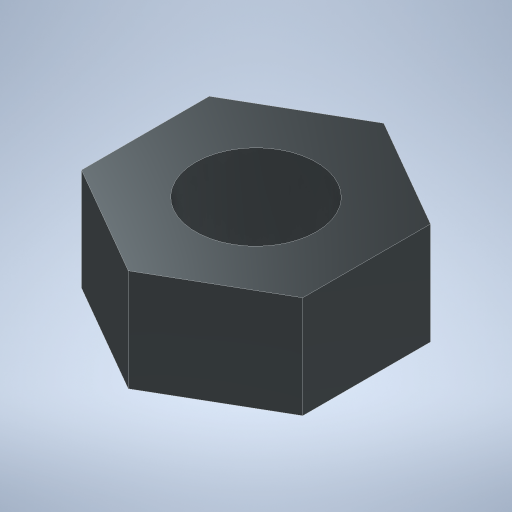
# Autodesk Inventor part: Threaded Rod nut
Saved by Autodesk Inventor 2024 (Build 280153000, 153)
## iProperties
Created: 2023-06-07
Part Number: Threaded Rod nut
Material: Generic
Document SubType Name: Modeling
Designer: 18179
Density: 1 g/cm^3
Appearance: Iron Gray
Author: 18179
Autodesk Inventor part; units mm, degrees
ref_plane "YZ Plane" through (0, 0, 0) normal (1, 0, 0) x (0, 1, 0)
ref_plane "XZ Plane" through (0, 0, 0) normal (0, 1, 0) x (-1, 0, 0)
ref_plane "XY Plane" through (0, 0, 0) normal (0, 0, 1) x (1, 0, 0)
sketch "Sketch1" plane through (0, 0, 0) normal (0, 1, 0) x (-1, 0, 0)
  line L0 (2.75, -1.5877) -> (0, -3.1754)
  line L1 (0, -3.1754) -> (-2.75, -1.5877)
  line L2 (-2.75, -1.5877) -> (-2.75, 1.5877)
  line L3 (-2.75, 1.5877) -> (0, 3.1754)
  line L4 (0, 3.1754) -> (2.75, 1.5877)
  line L5 (2.75, 1.5877) -> (2.75, -1.5877)
  circle A0 centre (0, 0) radius 1.5
  point P0 (2.75, 0)
  dimension "d0" = 2.75
  dimension "d1" = 3
  constraints: 12 end point, 2 coincident, 1 centre point, 1 midpoint, 13 other
  measures "d0" distance of point (2.75, 0) point (0, 0)
  measures "d1" diameter of A0
extrude "Extrusion1" add sketch "Sketch1" along normal blind 2.54
body "Solid1"
